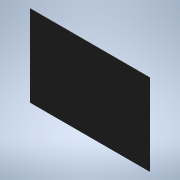
# Autodesk Inventor part: SP41V1 Goma Base
Saved by Autodesk Inventor 2021.2 (Build 252289000, 289)
## iProperties
Created: 2026-08-25
Part Number: SP41V1 Goma Base
Material: Rubber
Document SubType Name: Modeling
Designer: nelso
Density: 0.93 g/cm^3
Appearance: Rubber - Black
Author: nelso
Autodesk Inventor part; units mm, degrees
ref_plane "YZ Plane" through (0, 0, 0) normal (1, 0, 0) x (0, 1, 0)
ref_plane "XZ Plane" through (0, 0, 0) normal (0, 1, 0) x (-1, 0, 0)
ref_plane "XY Plane" through (0, 0, 0) normal (0, 0, 1) x (1, 0, 0)
sketch "Sketch1" plane through (0, 0, 0) normal (0, 1, 0) x (-1, 0, 0)
  line L0 (355, 241.5) -> (-355, 241.5)
  line L1 (-355, 241.5) -> (-355, -241.5)
  line L2 (-355, -241.5) -> (355, -241.5)
  line L3 (355, -241.5) -> (355, 241.5)
  line L4 (355, 241.5) -> (-355, -241.5) construction
  line L5 (-355, 241.5) -> (355, -241.5) construction
  point P0 (0, 0)
  dimension "d0" = 710
  dimension "d1" = 483
  constraints: 12 end point, 2 midpoint, 2 parallel, 1 horizontal, 1 perpendicular
  measures "d0" distance of L2.end L1.end
  measures "d1" distance of L1.end L0.end
extrude "Extrusion1" add sketch "Sketch1" along normal blind 3
body "Solid1"
